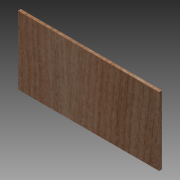
# Autodesk Inventor part: stand_bottom
Saved by Autodesk Inventor 2017 (Build 210142000, 142)
## iProperties
Created: 2018-10-12
Part Number: stand_bottom
Material: Wood (Birch)
Document SubType Name: Modeling
Designer: ari
Density: 0.55 g/cm^3
Appearance: Birch - Natural Polished
Author: ari
Autodesk Inventor part; units mm, degrees
ref_plane "YZ Plane" through (0, 0, 0) normal (1, 0, 0) x (0, 1, 0)
ref_plane "XZ Plane" through (0, 0, 0) normal (0, 1, 0) x (-1, 0, 0)
ref_plane "XY Plane" through (0, 0, 0) normal (0, 0, 1) x (1, 0, 0)
sketch "Sketch1" plane through (0, 0, 0) normal (0, 0, 1) x (1, 0, 0)
  line L0 (0, 0) -> (-250, 0)
  line L1 (-250, 0) -> (-250, 5)
  line L2 (-250, 5) -> (0, 5)
  line L3 (0, 5) -> (0, 0)
  dimension "d0" = 5
  dimension "d1" = 250
  constraints: 8 end point, 2 parallel, 1 horizontal, 1 perpendicular
  measures "d0" distance of L2.end L0.start
  measures "d1" distance of L0.start L0.end
extrude "Extrusion1" add sketch "Sketch1" along normal blind 121
body "Solid1"
